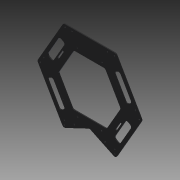
# Autodesk Inventor part: Bottom Plate
Saved by Autodesk Inventor 2015 (Build 190159000, 159)
## iProperties
Created: 2016-10-01
Part Number: Bottom Plate
Material: PVC, Unplasticized
Document SubType Name: Modeling
Designer: James Yelland
Density: 1.29 g/cm^3
Appearance: Smooth - White
Mass: 31.7822 g
Surface Area: 281.879 cm^2
Volume: 24.6374 cm^3
Author: James Yelland
Autodesk Inventor part; units mm, degrees
ref_plane "YZ Plane" through (0, 0, 0) normal (1, 0, 0) x (0, 1, 0)
ref_plane "XZ Plane" through (0, 0, 0) normal (0, 1, 0) x (-1, 0, 0)
ref_plane "XY Plane" through (0, 0, 0) normal (0, 0, 1) x (1, 0, 0)
sketch "Sketch1" plane through (0, 0, 0) normal (0, 1, 0) x (-1, 0, 0)
  line L0 (72.6878, -41.9663) -> (62.1878, -60.1529)
  line L1 (72.6878, -41.9663) -> (83.1878, -23.7798)
  line L2 (81.7237, -18.3157) -> (77.3936, -15.8157)
  line L3 (71.9295, -17.2797) -> (50.9295, -53.6529)
  line L4 (52.3936, -59.117) -> (56.7237, -61.617)
  arc A0 (56.7237, -61.617) -> (62.1878, -60.1529) centre (58.7237, -58.1529) ccw
  arc A1 (50.9295, -53.6529) -> (52.3936, -59.117) centre (54.3936, -55.6529) ccw
  arc A2 (77.3936, -15.8157) -> (71.9295, -17.2797) centre (75.3936, -19.2798) ccw
  arc A3 (83.1878, -23.7798) -> (81.7237, -18.3157) centre (79.7237, -21.7798) ccw
  line L5 (-72.6878, -41.9663) -> (-83.1878, -23.7798)
  line L6 (-72.6878, -41.9663) -> (-62.1878, -60.1529)
  line L7 (-56.7237, -61.617) -> (-52.3936, -59.117)
  line L8 (-50.9295, -53.6529) -> (-71.9294, -17.28)
  line L9 (-77.3936, -15.8157) -> (-81.7237, -18.3157)
  arc A4 (-81.7237, -18.3157) -> (-83.1878, -23.7798) centre (-79.7237, -21.7798) ccw
  arc A5 (-71.9294, -17.28) -> (-77.3936, -15.8157) centre (-75.3936, -19.2798) ccw
  arc A6 (-52.3936, -59.117) -> (-50.9295, -53.6529) centre (-54.3936, -55.6529) ccw
  arc A7 (-62.1878, -60.1529) -> (-56.7237, -61.617) centre (-58.7237, -58.1529) ccw
  line L10 (103.5566, -2.5) -> (54.8095, -86.9325)
  line L11 (-54.8095, -86.9325) -> (-103.5566, -2.5)
  line L12 (-103.5566, 2.5) -> (-53.9434, 88.4327)
  line L13 (-49.6132, 90.9327) -> (49.6132, 90.9327)
  line L14 (53.9434, 88.4327) -> (103.5566, 2.5)
  line L15 (2.1497, -66.9563) -> (48.3297, -88.9468)
  line L16 (-2.1497, -66.9563) -> (-48.3297, -88.9468)
  arc A8 (48.3297, -88.9468) -> (54.8095, -86.9325) centre (50.4794, -84.4325) ccw
  arc A9 (2.1497, -66.9563) -> (-2.1497, -66.9563) centre (0, -71.4706) ccw
  arc A10 (-54.8095, -86.9325) -> (-48.3297, -88.9468) centre (-50.4794, -84.4325) ccw
  arc A11 (-103.5566, 2.5) -> (-103.5566, -2.5) centre (-99.2265, 0) ccw
  arc A12 (-49.6132, 90.9327) -> (-53.9434, 88.4327) centre (-49.6132, 85.9327) ccw
  arc A13 (53.9434, 88.4327) -> (49.6132, 90.9327) centre (49.6132, 85.9327) ccw
  arc A14 (103.5566, -2.5) -> (103.5566, 2.5) centre (99.2265, 0) ccw
  circle A15 centre (49.6132, 85.9327) radius 1.6
  circle A16 centre (-49.6132, 85.9327) radius 1.6
  circle A17 centre (-99.2265, 0) radius 1.6
  circle A18 centre (99.2265, 0) radius 1.6
  circle A19 centre (-25, 62.282) radius 1.6
  circle A20 centre (25, 62.282) radius 1.6
  circle A21 centre (24, -57.282) radius 1.6
  circle A22 centre (-24, -57.282) radius 1.6
  line L17 (72.6878, 41.9663) -> (62.1878, 60.1529)
  line L18 (72.6878, 41.9663) -> (83.1878, 23.7798)
  line L19 (81.7237, 18.3157) -> (77.3936, 15.8157)
  line L20 (71.9295, 17.2797) -> (50.9295, 53.6529)
  line L21 (52.3936, 59.117) -> (56.7237, 61.617)
  arc A23 (62.1878, 60.1529) -> (56.7237, 61.617) centre (58.7237, 58.1529) ccw
  arc A24 (52.3936, 59.117) -> (50.9295, 53.6529) centre (54.3936, 55.6529) ccw
  arc A25 (71.9295, 17.2797) -> (77.3936, 15.8157) centre (75.3936, 19.2798) ccw
  arc A26 (81.7237, 18.3157) -> (83.1878, 23.7798) centre (79.7237, 21.7798) ccw
  arc A27 (-56.7237, 61.617) -> (-62.1878, 60.1529) centre (-58.7237, 58.1529) ccw
  line L22 (-56.7237, 61.617) -> (-52.3936, 59.117)
  arc A28 (-50.9295, 53.6529) -> (-52.3936, 59.117) centre (-54.3936, 55.6529) ccw
  line L23 (-72.6878, 41.9663) -> (-62.1878, 60.1529)
  line L24 (-50.9295, 53.6529) -> (-71.9294, 17.28)
  line L25 (-72.6878, 41.9663) -> (-83.1878, 23.7798)
  arc A29 (-83.1878, 23.7798) -> (-81.7237, 18.3157) centre (-79.7237, 21.7798) ccw
  line L26 (-77.3936, 15.8157) -> (-81.7237, 18.3157)
  arc A30 (-77.3936, 15.8157) -> (-71.9294, 17.28) centre (-75.3936, 19.2798) ccw
  circle A31 centre (50.4794, -84.4325) radius 1.45
  circle A32 centre (50.4794, -76.4325) radius 1.45
  circle A33 centre (-50.4794, -76.4325) radius 1.45
  circle A34 centre (-50.4794, -84.4325) radius 1.45
  circle A35 centre (-30.6147, -73.9104) radius 1.6
  circle A36 centre (30.6147, -73.9104) radius 1.6
  circle A37 centre (35.5991, 85.9437) radius 1.6
  circle A38 centre (-35.5945, 85.9327) radius 1.6
  circle A39 centre (92.2171, 12.1406) radius 1.6
  circle A40 centre (-92.2171, 12.1406) radius 1.6
  line L27 (-62.0082, -23.9647) -> (-51.7576, -41.7179)
  line L28 (-51.7576, -41.7179) -> (-53.9226, -42.9679)
  line L29 (-53.9226, -42.9679) -> (-64.1732, -25.2148)
  line L30 (-64.1732, -25.2148) -> (-62.0082, -23.9647)
  line L31 (51.7581, -41.7183) -> (62.0075, -23.9645)
  line L32 (62.0075, -23.9645) -> (64.1726, -25.2144)
  line L33 (64.1726, -25.2144) -> (53.9232, -42.9683)
  line L34 (53.9232, -42.9683) -> (51.7581, -41.7183)
  line L35 (62.0082, 23.9647) -> (51.7576, 41.7179)
  line L36 (51.7576, 41.7179) -> (53.9226, 42.9679)
  line L37 (53.9226, 42.9679) -> (64.1732, 25.2148)
  line L38 (64.1732, 25.2148) -> (62.0082, 23.9647)
  line L39 (-51.7581, 41.7183) -> (-62.0075, 23.9645)
  line L40 (-62.0075, 23.9645) -> (-64.1726, 25.2144)
  line L41 (-64.1726, 25.2144) -> (-53.9232, 42.9683)
  line L42 (-53.9232, 42.9683) -> (-51.7581, 41.7183)
  arc A41 (31.3397, -49.282) -> (35.6699, -46.782) centre (31.3397, -44.282) ccw
  line L43 (31.3397, -49.282) -> (-31.3397, -49.282)
  arc A42 (-35.6699, -46.782) -> (-31.3397, -49.282) centre (-31.3397, -44.282) ccw
  line L44 (-35.6699, -46.782) -> (-61.2361, -2.5)
  arc A43 (-61.2361, 2.5) -> (-61.2361, -2.5) centre (-56.906, 0) ccw
  line L45 (-61.2361, 2.5) -> (-32.7831, 51.782)
  arc A44 (-28.453, 54.282) -> (-32.7831, 51.782) centre (-28.453, 49.282) ccw
  line L46 (-28.453, 54.282) -> (28.453, 54.282)
  arc A45 (32.7831, 51.782) -> (28.453, 54.282) centre (28.453, 49.282) ccw
  line L47 (32.7831, 51.782) -> (61.2361, 2.5)
  arc A46 (61.2361, -2.5) -> (61.2361, 2.5) centre (56.906, 0) ccw
  line L48 (61.2361, -2.5) -> (35.6699, -46.782)
  point P0 (60.1878, -63.617)
  point P1 (85.1878, -20.3157)
  point P2 (73.9295, -13.8157)
  point P3 (48.9295, -57.117)
  point P4 (-85.1878, -20.3157)
  point P5 (-60.1878, -63.617)
  point P6 (-48.9295, -57.117)
  point P7 (-73.9295, -13.8157)
  point P8 (105, 0)
  point P9 (52.5, -90.9327)
  point P10 (-105, 0)
  point P11 (-52.5, 90.9327)
  point P12 (52.5, 90.9327)
  point P13 (60.1878, 63.617)
  point P14 (85.1878, 20.3157)
  point P15 (73.9295, 13.8157)
  point P16 (48.9295, 57.117)
  point P17 (-48.9295, 57.117)
  point P18 (-60.1878, 63.617)
  point P19 (-73.9295, 13.8157)
  point P20 (-85.1878, 20.3157)
  dimension "d11" = 360
  dimension "d30" = 360
  dimension "d90" = 360
  dimension "d136" = 360
  constraints: 98 end point, 58 point on circle, 53 centre point, 41 point on line, 6 coincident
extrude "Extrusion1" add sketch "Sketch1" along normal blind 2
body "Solid1"
